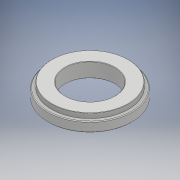
# Autodesk Inventor part: IGX間隔環
Saved by Autodesk Inventor 2018 (Build 220112000, 112)
## iProperties
Created: 2025-11-25
Part Number: IGX間隔環
Material: 一般
Document SubType Name: Modeling
Designer: User
Density: 1 g/cm^3
Appearance: 預設
Author: User
Autodesk Inventor part; units mm, degrees
ref_plane "YZ Plane" through (0, 0, 0) normal (1, 0, 0) x (0, 1, 0)
ref_plane "XZ Plane" through (0, 0, 0) normal (0, 1, 0) x (-1, 0, 0)
ref_plane "XY Plane" through (0, 0, 0) normal (0, 0, 1) x (1, 0, 0)
sketch "草圖1" plane through (0, 0, 0) normal (0, 0, 1) x (1, 0, 0)
  circle A0 centre (0, 0) radius 18.05
  circle A1 centre (0, 0) radius 30.65
  dimension "d0" = 36.1
  dimension "d1" = 61.3
  constraints: 2 centre point, 2 coincident
  measures "d0" diameter of A0
  measures "d1" diameter of A1
extrude "擠出1" add sketch "草圖1" along normal blind 10.61
sketch "草圖2" plane through (0, 0, 10.61) normal (0, 0, 1) x (1, 0, 0)
  circle A0 centre (0, 0) radius 28
  circle A1 centre (0, 0) radius 39.6506
  dimension "d4" = 56
  constraints: 2 centre point, 2 coincident
  measures "d4" diameter of A0
extrude "擠出2" cut sketch "草圖2" against normal blind 3.6
chamfer "倒角1" distance 0.3 angle 45 1 edges at (-18.05, 0, 0)
chamfer "倒角2" distance 0.5 angle 45 1 edges at (-30.65, 0, 0)
chamfer "倒角3" distance 0.5 angle 45 1 edges at (-30.65, 0, 7.01)
fillet "圓角1" radius 0.25 1 edges at (-28, 0, 10.61)
chamfer "倒角4" distance 0.3 angle 45 1 edges at (-18.05, 0, 10.61)
